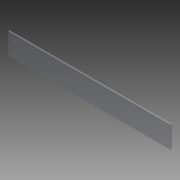
# Autodesk Inventor part: Polycarbonate Sheet
Saved by Autodesk Inventor 2014 (Build 180170000, 170)
## iProperties
Created: 2014-01-20
Part Number: Polycarbonate Sheet
Material: Polycarbonate, Clear
Document SubType Name: Modeling
Designer: Andrew Toennies
Mass: 73.5366 g
Surface Area: 415.09 cm^2
Volume: 61.2805 cm^3
Density: 1.2 g/cm^3
Appearance: Polycarbonate - Clear
Author: Andrew Toennies
Autodesk Inventor part; units mm, degrees
ref_plane "YZ Plane" through (0, 0, 0) normal (1, 0, 0) x (0, 1, 0)
ref_plane "XZ Plane" through (0, 0, 0) normal (0, 1, 0) x (-1, 0, 0)
ref_plane "XY Plane" through (0, 0, 0) normal (0, 0, 1) x (1, 0, 0)
sketch "Sketch1" plane through (0, 0, 0) normal (0, 0, 1) x (1, 0, 0)
  line L0 (0, 0) -> (381, 0)
  line L1 (381, 0) -> (381, 50.8)
  line L2 (381, 50.8) -> (0, 50.8)
  line L3 (0, 50.8) -> (0, 0)
  circle A0 centre (12.7, 12.7) radius 2.0701
  circle A1 centre (12.7, 38.1) radius 2.0701
  circle A2 centre (368.3, 12.7) radius 2.0701
  circle A3 centre (368.3, 38.1) radius 2.0701
  dimension "d0" = 50.8
  dimension "d1" = 381
  dimension "d2" = 4.1402
  dimension "d3" = 12.7
  dimension "d4" = 12.7
  dimension "d7" = 25.4
  dimension "d10" = 355.6
  constraints: 8 end point, 4 centre point, 2 horizontal, 2 parallel, 1 perpendicular, 1 vertical, 6 other
  measures "d0" distance of L2.end L0.start
  measures "d1" distance of L1.end L2.end
  measures "d2" diameter of A0
  measures "d3" distance from line of L0 A0.centre
  measures "d4" distance from line of L3 A0.centre
  measures "d7" distance of A0.centre A1.centre
  measures "d10" distance of A0.centre A2.centre
extrude "Extrusion1" add sketch "Sketch1" along normal blind 3.175
body "Solid1"
